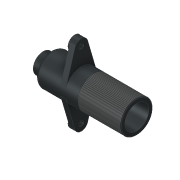
# Autodesk Inventor part: 05.01.003
Saved by Autodesk Inventor 2019.3 (Build 233278000, 278)
## iProperties
Created: 2018-07-09
Part Number: 05.01.003
Material: Чугун, серый
Document SubType Name: Modeling
Designer: MSI-PC
Mass: 909.454 g
Surface Area: 435.812 cm^2
Volume: 127.196 cm^3
Density: 7.15 g/cm^3
Appearance: Чугун серый
Description: Корпус
Author: MSI-PC
Title: Корпус
Autodesk Inventor part; units mm, degrees
ref_plane "YZ Plane" through (0, 0, 0) normal (1, 0, 0) x (0, 1, 0)
ref_plane "XZ Plane" through (0, 0, 0) normal (0, 1, 0) x (-1, 0, 0)
sketch "Эскиз1" plane through (0, 0, 0) normal (0, 0, 1) x (1, 0, 0)
  line L0 (0, 0) -> (140, 0)
  line L1 (0, 0) -> (0, 15)
  line L2 (0, 15) -> (12, 15)
  line L3 (12, 15) -> (12, 24)
  line L4 (12, 24) -> (140, 24)
  line L5 (140, 24) -> (140, 0)
  dimension "d1" = 30
  dimension "d2" = 48
  dimension "d3" = 12
  dimension "d4" = 140
  constraints: 12 end point, 4 perpendicular, 1 horizontal, 1 vertical
  measures "d1" diameter of L2 L0
  measures "d2" diameter of L4 L0
  measures "d3" distance between parallel lines of L3 L1
  measures "d4" distance between parallel lines of L5 L1
revolve "Вращение1" add sketch "Эскиз1" angle 360 about axis through (0, 0, 0) along (1, 0, 0)
ref_plane "РабПлоскость1" through (57, 0, 0) normal (1, 0, 0) x (0, 0, -1)
sketch "Эскиз2" plane through (57, 0, 0) normal (1, 0, 0) x (0, 0, -1)
  arc A0 (0, 40) -> (9.6, 52.8) centre (0, 50) ccw
  circle A1 centre (0, 0) radius 24 projected
  line L0 (-23.04, 6.72) -> (-9.6, 52.8)
  line L1 (0, -43.1124) -> (0, 90.6743) projected
  line L2 (23.04, 6.72) -> (9.6, 52.8)
  circle A2 centre (0, 50) radius 4
  arc A3 (23.04, 6.72) -> (-23.04, 6.72) centre (0, 0) ccw
  arc A4 (-9.6, 52.8) -> (0, 40) centre (0, 50) ccw
  arc A5 (9.6, 52.8) -> (-9.6, 52.8) centre (0, 50) ccw
  point P0 (0, 0)
  dimension "d7" = 20
  dimension "d8" = 8
  dimension "d13" = 50
  constraints: 8 point on circle, 5 centre point, 4 end point, 4 tangent, 2 symmetric about line, 1 coincident, 1 point on line, 1 vertical alignment, 3 other
  measures "d7" diameter of A0
  measures "d8" diameter of A2
  measures "d13" distance of point (0, 0) A0.centre
extrude "Выдавливание1" add sketch "Эскиз2" against normal blind 8 contours L1 A2 A5 A0 | A0 L2 A1 L1 | A4 A5 L1 A2 | L1 A1 L0 A4
extrude "Выдавливание2" add sketch "Эскиз2" against normal blind 10 contours L1 A2 A5 A0 | A4 A5 L1 A2
mirror "Зеркальное отражение1" about plane through (0, 0, 0) normal (0, 1, 0) of "Выдавливание1", "Выдавливание2"
sketch "Эскиз3" plane through (140, 0, 0) normal (1, 0, 0) x (0, 0, -1)
  circle A0 centre (0, 0) radius 24 projected
  constraints: 1 coincident
hole "Отверстие1" at (140, 0, 0) direction (-1, 0, 0) diameter 36 depth 120
sketch "Эскиз4" plane through (0, 0, 0) normal (-1, 0, 0) x (0, 0, 1)
  line L0 (9, 9) -> (9, -9)
  line L1 (9, -9) -> (-9, -9)
  line L2 (-9, -9) -> (-9, 9)
  line L3 (-9, 9) -> (9, 9)
  point P0 (0, 0)
  point P1 (0, 0)
  dimension "d21" = 18
  constraints: 8 end point, 1 coincident, 1 horizontal, 9 other
  measures "d21" distance of L0.start L0.end
extrude "Выдавливание3" cut sketch "Эскиз4" against normal up to surface (20 mm away)
thread "Резьба1" size "M48x1.5" class "6g" standard "ISO Metric profile" length 64
fillet "Сопряжение1" radius 5 1 edges at (12, -24, 0)
chamfer "Фаска1" distance 1 angle 45 1 edges at (140, -24, 0)
